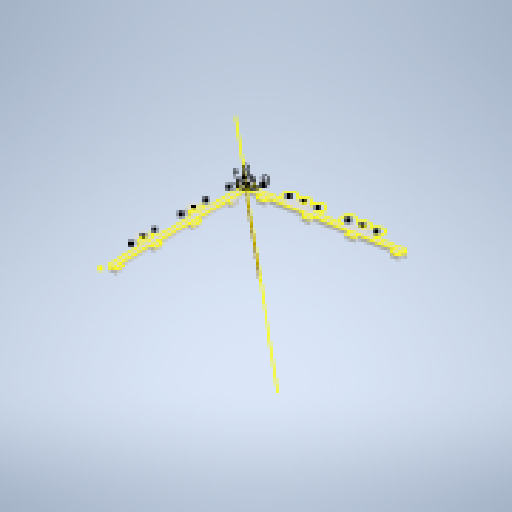
# Autodesk Inventor part: крепежная деталь для клюва
Saved by Autodesk Inventor 2023.2 (Build 272271030, 271C)
## iProperties
Created: 2024-02-14
Part Number: крепежная деталь для клюва
Material: Типовые
Document SubType Name: Modeling
Designer: liza
Density: 1 g/cm^3
Appearance: По умолчанию
Author: liza
Autodesk Inventor part; units mm, degrees
ref_plane "YZ Plane" through (0, 0, 0) normal (1, 0, 0) x (0, 1, 0)
ref_plane "XZ Plane" through (0, 0, 0) normal (0, 1, 0) x (-1, 0, 0)
ref_plane "XY Plane" through (0, 0, 0) normal (0, 0, 1) x (1, 0, 0)
sketch "Эскиз1" plane through (0, 0, 0) normal (1, 0, 0) x (0, 1, 0)
  line L0 (0, 0) -> (3, 0)
  line L1 (3, 0) -> (3, -95)
  line L2 (3, -95) -> (0, -95)
  line L3 (0, -95) -> (0, 0)
  dimension "d0" = 95
  dimension "d2" = 3
  constraints: 8 end point, 2 parallel, 1 horizontal, 1 perpendicular
  measures "d0" distance of L0.end L1.end
  measures "d2" distance of L1.end L2.end
extrude "Выдавливание1" add sketch "Эскиз1" along normal blind 3
sketch "Эскиз2" plane through (3, 0, 0) normal (1, 0, 0) x (0, 0, -1)
  line L0 (4.09, 3) -> (9.09, 3)
  line L1 (9.09, 3) -> (9.09, 0)
  line L2 (9.09, 0) -> (4.09, 0)
  line L3 (4.09, 0) -> (4.09, 3)
  line L4 (95, 3) -> (0, 3) projected
  line L5 (3.7261, 3) -> (3.7261, 3)
  line L6 (6.59, 0) -> (6.59, 0)
  line L7 (0, 0) -> (95, 0) projected
  line L8 (0, 3) -> (0, 0) projected
  dimension "d5" = 5
  dimension "d6" = 3
  dimension "d12" = 4.09
  constraints: 12 end point, 4 parallel, 3 point on line, 2 perpendicular, 1 horizontal, 1 midpoint
  measures "d5" distance of L0.start L0.end
  measures "d6" distance of L0.end L1.end
  measures "d12" distance between parallel lines of L8 L3
extrude "Выдавливание2" add sketch "Эскиз2" along normal blind 3 contours L0 L1 L2 L3
pattern_linear "Прямоуг.массив1" count 4 spacing 25.2 along (0, 0, -1) of "Выдавливание2"
sketch "Эскиз3" plane through (0, 3, 0) normal (0, 1, 0) x (1, 0, 0)
  line L0 (0, 95) -> (0, 0) construction
  line L1 (0, 27.6667) -> (0, 35.6667)
  line L2 (0, 35.6667) -> (-8, 35.6667)
  line L3 (-8, 35.6667) -> (-8, 27.6667)
  line L4 (-8, 27.6667) -> (0, 27.6667)
  circle A0 centre (-4, 31.6667) radius 1.45
  line L5 (-8, 27.6667) -> (0, 35.6667) construction
  line L6 (0, 0) -> (-35.0578, 0) construction
  line L7 (-35.0578, 0) -> (-35.0578, 31.6667) construction
  line L8 (-35.0578, 31.6667) -> (-35.0578, 63.3333) construction
  line L9 (-35.0578, 63.3333) -> (-35.0578, 95) construction
  line L10 (-35.0578, 95) -> (0, 95) construction
  line L11 (-4, 31.6667) -> (-35.0578, 31.6667) construction
  dimension "d13" = 2.9
  dimension "d14" = 8
  dimension "d24" = 31.6667
  constraints: 22 end point, 4 point on line, 3 equal length, 3 perpendicular, 2 horizontal, 2 parallel, 1 centre point, 1 coincident, 1 midpoint
  measures "d13" diameter of A0
  measures "d14" distance of L2.end L3.end
  measures "d24" distance of L7.end L8.end
extrude "Выдавливание3" add sketch "Эскиз3" against normal blind 3
fillet "Сопряжение1" radius 4 4 edges at (0, 1.5, -27.6667) (-8, 1.5, -27.6667) (-8, 1.5, -35.6667) (0, 1.5, -35.6667)
pattern_linear "Прямоуг.массив2" count 2 spacing 33.3333 along (0, 0, -1) of "Сопряжение1", "Выдавливание3"
ref_plane "РабПлоскость1" through (0, 0, -95) normal (-0.6427876, 0, 0.7660444) x (0, 1, 0)
sketch "Эскиз4" plane through (0, 3, 0) normal (0, 1, 0) x (1, 0, 0)
  line L0 (3, 2.4447) -> (0, 5.3135)
  line L1 (0, 5.3135) -> (0, 0)
  line L2 (3, 0) -> (3, 4.09) projected
  line L3 (0, 0) -> (3, 0)
  line L4 (3, 0) -> (3, 2.4447)
  constraints: 8 end point, 1 collinear, 1 perpendicular, 1 vertical
extrude "Выдавливание4" cut sketch "Эскиз4" against normal blind 3
mirror "Зеркальное отражение1" about plane through (0, 0, -95) normal (-0.6427876, 0, 0.7660444)
sketch "Эскиз5" plane through (6, 3, -4.09) normal (0, 1, 0) x (1, 0, 0)
  line L0 (-6, 90.91) -> (-6, 68.91) construction
  line L1 (-6.9861, 96.959) -> (-12.1284, 90.8307)
  line L2 (-12.1284, 90.8307) -> (-6, 85.6884)
  line L3 (-6, 85.6884) -> (-0.8577, 91.8167)
  line L4 (-0.8577, 91.8167) -> (-6.9861, 96.959)
  line L5 (-6.9861, 96.959) -> (-6, 85.6884) construction
  line L6 (-12.1284, 90.8307) -> (-0.8577, 91.8167) construction
  circle A0 centre (-6.493, 91.3237) radius 1.45
  line L7 (117.7825, -12.9558) -> (-44.6867, 123.372) projected
  line L8 (-6, 90.91) -> (15.6658, 94.7303) construction
  point P0 (-6, -4.09)
  point P1 (-9.5572, 93.8948)
  point P2 (-3.4288, 88.7525)
  dimension "d29" = 2.9
  dimension "d30" = 8
  constraints: 12 end point, 4 midpoint, 3 point on line, 2 parallel, 2 perpendicular, 1 centre point, 1 coincident
  measures "d29" diameter of A0
  measures "d30" distance of L1.start L1.end
extrude "Выдавливание5" add sketch "Эскиз5" against normal blind 3 contours L4 L3 L7 A0 L1 | L7 A0 L3 L2 L1
extrude "Выдавливание6" cut sketch "Эскиз5" against normal blind 3 contours L7 A0 | A0 L7
fillet "Сопряжение2" radius 4 4 edges at (-6.1284, 1.5, -94.9207) (0, 1.5, -89.7784) (-0.9861, 1.5, -101.049) (5.1423, 1.5, -95.9067)
sketch "Эскиз6" plane through (6, 3, -4.09) normal (0, 1, 0) x (1, 0, 0)
  circle A0 centre (-6.493, 91.3237) radius 1.45 projected
  arc A1 (-9.0642, 88.2595) -> (-3.9219, 94.3879) centre (-6.493, 91.3237) ccw projected
  line L0 (-9.0642, 88.2595) -> (-7.4288, 86.8873) projected
  arc A2 (-6, 83.8231) -> (-7.4288, 86.8873) centre (-10, 83.8231) ccw projected
  line L1 (-6, 83.8231) -> (-6, 68.91) projected
  arc A3 (-10, 64.91) -> (-6, 68.91) centre (-10, 68.91) ccw projected
  arc A4 (-10, 56.91) -> (-10, 64.91) centre (-10, 60.91) ccw projected
  arc A5 (-6, 52.91) -> (-10, 56.91) centre (-10, 52.91) ccw projected
  line L2 (-6, 52.91) -> (-6, 35.5767) projected
  arc A6 (-10, 31.5767) -> (-6, 35.5767) centre (-10, 35.5767) ccw projected
  arc A7 (-10, 23.5767) -> (-10, 31.5767) centre (-10, 27.5767) ccw projected
  arc A8 (-6, 19.5767) -> (-10, 23.5767) centre (-10, 19.5767) ccw projected
  line L3 (-6, 19.5767) -> (-6, 1.2235) projected
  line L4 (-6, 1.2235) -> (-3, -1.6453) projected
  line L5 (-3, 0) -> (-3, -1.6453) projected
  line L6 (-3, 0) -> (0, 0) projected
  line L7 (0, 5) -> (0, 0) projected
  line L8 (-3, 5) -> (0, 5) projected
  line L9 (-3, 25.2) -> (-3, 5) projected
  line L10 (-3, 25.2) -> (0, 25.2) projected
  line L11 (0, 30.2) -> (0, 25.2) projected
  line L12 (-3, 30.2) -> (0, 30.2) projected
  line L13 (-3, 50.4) -> (-3, 30.2) projected
  line L14 (-3, 50.4) -> (0, 50.4) projected
  line L15 (0, 55.4) -> (0, 50.4) projected
  line L16 (-3, 55.4) -> (0, 55.4) projected
  line L17 (-3, 75.6) -> (-3, 55.4) projected
  line L18 (-3, 88.3927) -> (-3, 80.6) projected
  line L19 (-3, 88.3927) -> (4.6743, 89.7459) projected
  line L20 (4.6743, 89.7459) -> (5.1953, 86.7915) projected
  line L21 (5.1953, 86.7915) -> (10.1193, 87.6597) projected
  line L22 (9.5984, 90.6141) -> (10.1193, 87.6597) projected
  line L23 (9.5984, 90.6141) -> (29.4915, 94.1218) projected
  line L24 (29.4915, 94.1218) -> (30.0124, 91.1674) projected
  line L25 (30.0124, 91.1674) -> (34.9365, 92.0356) projected
  line L26 (34.4155, 94.9901) -> (34.9365, 92.0356) projected
  line L27 (34.4155, 94.9901) -> (54.3086, 98.4978) projected
  line L28 (54.3086, 98.4978) -> (54.8296, 95.5433) projected
  line L29 (54.8296, 95.5433) -> (59.7536, 96.4116) projected
  line L30 (59.2327, 99.366) -> (59.7536, 96.4116) projected
  line L31 (59.2327, 99.366) -> (79.1258, 102.8737) projected
  line L32 (79.1258, 102.8737) -> (79.6467, 99.9193) projected
  line L33 (79.6467, 99.9193) -> (84.5708, 100.7875) projected
  line L34 (84.0498, 103.7419) -> (84.5708, 100.7875) projected
  line L35 (84.0498, 103.7419) -> (85.6701, 104.0276) projected
  line L36 (82.3239, 106.4839) -> (85.6701, 104.0276) projected
  line L37 (64.2496, 103.2969) -> (82.3239, 106.4839) projected
  arc A9 (64.2496, 103.2969) -> (59.6158, 106.5415) centre (63.555, 107.2361) ccw projected
  arc A10 (59.6158, 106.5415) -> (51.7373, 105.1524) centre (55.6766, 105.8469) ccw projected
  arc A11 (51.7373, 105.1524) -> (48.4927, 100.5185) centre (47.7981, 104.4578) ccw projected
  line L38 (31.4227, 97.5086) -> (48.4927, 100.5185) projected
  arc A12 (31.4227, 97.5086) -> (26.7889, 100.7533) centre (30.7281, 101.4479) ccw projected
  arc A13 (26.7889, 100.7533) -> (18.9104, 99.3641) centre (22.8496, 100.0587) ccw projected
  arc A14 (18.9104, 99.3641) -> (15.6658, 94.7303) centre (14.9712, 98.6695) ccw projected
  line L39 (0.9792, 92.1406) -> (15.6658, 94.7303) projected
  arc A15 (-2.2865, 93.0157) -> (0.9792, 92.1406) centre (0.2846, 96.0799) ccw projected
  line L40 (-2.2865, 93.0157) -> (-3.9219, 94.3879) projected
  circle A16 centre (-10, 27.5767) radius 1.45 projected
  circle A17 centre (-10, 60.91) radius 1.45 projected
  circle A18 centre (55.6766, 105.8469) radius 1.45 projected
  circle A19 centre (22.8496, 100.0587) radius 1.45 projected
  line L41 (-3, 75.6) -> (0, 75.6) projected
  line L42 (-3, 75.6) -> (-3, 80.6) projected
  line L43 (8.7433, 95.4634) -> (3.8193, 94.5951) projected
  line L44 (33.5605, 99.8393) -> (28.6364, 98.9711) projected
  line L45 (58.3776, 104.2152) -> (53.4536, 103.347) projected
  line L46 (83.1948, 108.5912) -> (78.2707, 107.7229) projected
  line L47 (-3, 50.4) -> (-3, 55.4) projected
  line L48 (-3, 25.2) -> (-3, 30.2) projected
  line L49 (-3, 0) -> (-3, 5) projected
  point P0 (-6, -4.09)
  constraints: 20 centre point
